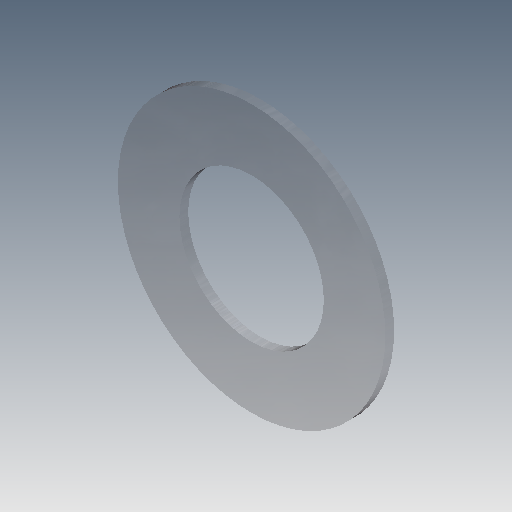
# Autodesk Inventor part: 軸受けワッシャC_ダブルスラスト用(t2_ジュラコン)
Saved by Autodesk Inventor 2019.4 (Build 234330000, 330)
## iProperties
Created: 2018-08-09
Part Number: 軸受けワッシャC_ダブルスラスト用(t2_ジュラコン)
Material: ポリカーボネート、クリア
Document SubType Name: Modeling
Designer: Owner
Mass: 1.69652 g
Surface Area: 23.0819 cm^2
Volume: 1.41377 cm^3
Density: 1.2 g/cm^3
Appearance: ポリカーボネート - クリア
Author: Owner
Autodesk Inventor part; units mm, degrees
ref_plane "YZ Plane" through (0, 0, 0) normal (1, 0, 0) x (0, 1, 0)
ref_plane "XZ Plane" through (0, 0, 0) normal (0, 1, 0) x (-1, 0, 0)
ref_plane "XY Plane" through (0, 0, 0) normal (0, 0, 1) x (1, 0, 0)
sketch "スケッチ1" plane through (0, 0, 0) normal (0, 0, 1) x (1, 0, 0)
  circle A0 centre (0, 0) radius 11.5 projected
  circle A1 centre (-13.5, -1.2593) radius 1.1 construction
  circle A2 centre (13.5, -1.2593) radius 1.1 construction
  circle A3 centre (0, 0) radius 20.5 projected
  circle A4 centre (0, 0) radius 21.3
  circle A5 centre (13.5, -1.2593) radius 1.1 construction
  circle A6 centre (-13.5, -1.2593) radius 1.1 construction
  circle A7 centre (0, 0) radius 18.011 construction
  line L0 (0, 0) -> (0, 18.011) construction
  circle A8 centre (0, -17.25) radius 0.8 construction
  circle A9 centre (0, 17.25) radius 0.8 construction
  circle A10 centre (17.25, 0) radius 0.8 construction
  circle A11 centre (-17.25, 0) radius 0.8 construction
  point P0 (0, 0)
  dimension "d0" = 42.6
  constraints: 2 end point, 1 centre point, 1 coincident, 1 vertical, 1 vertical alignment, 2 other
  measures "d0" diameter of A4
extrude "押し出し2" add sketch "スケッチ1" along normal blind 1.4 contours A3 | A4
